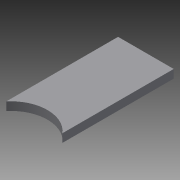
# Autodesk Inventor part: WingStiffener
Saved by Autodesk Inventor 2016 (Build 200138000, 138)
## iProperties
Created: 2015-05-10
Part Number: WingStiffener
Material: Generic
Document SubType Name: Modeling
Designer: Erin
Density: 1 g/cm^3
Appearance: Default
Author: Erin
Autodesk Inventor part; units mm, degrees
ref_plane "YZ Plane" through (0, 0, 0) normal (1, 0, 0) x (0, 1, 0)
ref_plane "XZ Plane" through (0, 0, 0) normal (0, 1, 0) x (-1, 0, 0)
ref_plane "XY Plane" through (0, 0, 0) normal (0, 0, 1) x (1, 0, 0)
sketch "Sketch1" plane through (0, 0, 0) normal (0, 0, 1) x (1, 0, 0)
  line L0 (-10, -4.7402) -> (10, -4.7402)
  line L1 (10, -4.7402) -> (10, -24.7402)
  line L2 (-10, -24.9327) -> (-10, -4.7402)
  arc A0 (10, -24.7402) -> (-10, -24.9327) centre (0.0817, -33.3215) ccw
  line L3 (-10, -4.7402) -> (10, -4.7402)
  line L4 (10, -4.7402) -> (10, 15.2598)
  line L5 (10, 15.2598) -> (-10, 15.2598)
  line L6 (-10, 15.2598) -> (-10, -4.7402)
  point P0 (0, 0)
  dimension "d0" = 20
  dimension "d1" = 20
  dimension "d2" = 20
  constraints: 14 end point, 3 parallel, 2 horizontal, 2 perpendicular, 2 point on circle, 1 centre point
  measures "d0" distance of L1.end L0.end
  measures "d1" distance between parallel lines of L1 L2
  measures "d2" distance of L3.end L4.end
extrude "Extrusion1" add sketch "Sketch1" along normal blind 3
body "Solid1"
